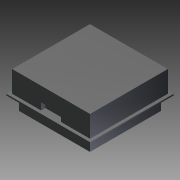
# Autodesk Inventor part: UB216SKG035D-1JBd_cap
Saved by Autodesk Inventor 2015 SP1 (Build 190203100, 203)
## iProperties
Category: Electrical
Company: Autodesk Inc.
Created: 2014-12-15
Part Number: UB216SKG035D-1JBd_cap
Catalog Web Link: http://www.nkkswitches.com/
Description: Low Profile Pushbuttons_diffuser_cap-Illuminated Pushbuttons - Series UB2
Vendor: NKK Switches
Document SubType Name: Modeling
Designer: Autodesk Inc.
Manufacturer: NKKSWITCHES
Mass: 1.18879 g
Surface Area: 8.09804 cm^2
Volume: 1.18879 cm^3
Density: 1 g/cm^3
Material: Generic
Appearance: PSOLRGB-192-192-192
Title: UB216SKG035D-1JBd_cap
Author: Autodesk Inc.
Autodesk Inventor part; units mm, degrees
sketch "Sketch_1" plane through (0, 0, 0) normal (0, 1, 0) x (-1, 0, 0)
  line L0 (7.5057, 7.5057) -> (-7.5057, 7.5057)
  line L1 (-7.5057, 7.5057) -> (-7.5057, -7.5057)
  line L2 (-7.5057, -7.5057) -> (7.5057, -7.5057)
  line L3 (7.5057, -7.5057) -> (7.5057, 7.5057)
  constraints: 8 end point
extrude "Extrusion1" add sketch "Sketch_1" along normal blind 4.0894
sketch "Sketch_2" plane through (0, 0.254, 0) normal (0, 1, 0) x (1, 0, 0)
  line L0 (-7.62, -7.62) -> (7.62, -7.62)
  line L1 (7.62, -7.62) -> (7.62, 7.62)
  line L2 (7.62, 7.62) -> (-7.62, 7.62)
  line L3 (-7.62, 7.62) -> (-7.62, -7.62)
  line L4 (-6.9723, -6.9723) -> (6.9723, -6.9723)
  line L5 (6.9723, -6.9723) -> (6.9723, 6.9723)
  line L6 (6.9723, 6.9723) -> (-6.9723, 6.9723)
  line L7 (-6.9723, 6.9723) -> (-6.9723, -6.9723)
  constraints: 16 end point
extrude "Extrusion2" cut sketch "Sketch_2" along normal blind 6.35
sketch "Sketch_4" plane through (0, 0, 6.9723) normal (0, 0, 1) x (1, 0, 0)
  line L0 (-1.778, 0.254) -> (1.778, 0.254)
  line L1 (1.778, 0.254) -> (1.778, 1.524)
  line L2 (1.778, 1.524) -> (-1.778, 1.524)
  line L3 (-1.778, 1.524) -> (-1.778, 0.254)
  constraints: 8 end point
extrude "Extrusion3" cut sketch "Sketch_4" against normal blind 0.762
sketch "Sketch_6" plane through (0, 0, 0) normal (0, 1, 0) x (-1, 0, 0)
  line L0 (6.35, 6.35) -> (-6.35, 6.35)
  line L1 (-6.35, 6.35) -> (-6.35, -6.35)
  line L2 (-6.35, -6.35) -> (6.35, -6.35)
  line L3 (6.35, -6.35) -> (6.35, 6.35)
  constraints: 8 end point
extrude "Extrusion4" add sketch "Sketch_6" against normal blind 2.413
ref_plane "diffuser_to_body_XY" through (0, 0, 0) normal (0, 1, 0) x (1, 0, 0)
ref_plane "diffuser_to_body_YZ" through (0, 0, 0) normal (1, 0, 0) x (0, 0, -1)
ref_plane "diffuser_to_body_ZX" through (0, 0, 0) normal (0, 0, -1) x (0, 1, 0)
ref_plane "diffuser_to_body_green_XY" through (3.7529, 0, 0) normal (0, 1, 0) x (1, 0, 0)
ref_plane "diffuser_to_body_green_YZ" through (3.7529, 0, 0) normal (1, 0, 0) x (0, 0, -1)
ref_plane "diffuser_to_body_green_ZX" through (3.7529, 0, 0) normal (0, 0, -1) x (0, 1, 0)
ref_plane "diffuser_to_body_red_XY" through (-3.7529, 0, 0) normal (0, 1, 0) x (1, 0, 0)
ref_plane "diffuser_to_body_red_YZ" through (-3.7529, 0, 0) normal (1, 0, 0) x (0, 0, -1)
ref_plane "diffuser_to_body_red_ZX" through (-3.7529, 0, 0) normal (0, 0, -1) x (0, 1, 0)
body "Solid1"
